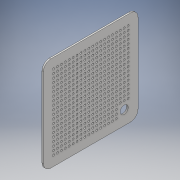
# Autodesk Inventor part: ExtrusionFrontpanel
Saved by Autodesk Inventor 2017 (Build 210142000, 142)
## iProperties
Created: 2019-06-19
Part Number: ExtrusionFrontpanel
Material: Generic
Document SubType Name: Modeling
Designer: DDeGo
Density: 1 g/cm^3
Appearance: Default
Author: DDeGo
Autodesk Inventor part; units mm, degrees
ref_plane "YZ Plane" through (0, 0, 0) normal (1, 0, 0) x (0, 1, 0)
ref_plane "XZ Plane" through (0, 0, 0) normal (0, 1, 0) x (-1, 0, 0)
ref_plane "XY Plane" through (0, 0, 0) normal (0, 0, 1) x (1, 0, 0)
sketch "Sketch1" plane through (0, 0, 0) normal (1, 0, 0) x (0, 1, 0)
  line L0 (0, 15) -> (160, 15)
  line L1 (175, 0) -> (175, -160)
  line L2 (160, -175) -> (0, -175)
  line L3 (-15, -160) -> (-15, 0)
  arc A0 (175, 0) -> (160, 15) centre (160, 0) ccw
  arc A1 (160, -175) -> (175, -160) centre (160, -160) ccw
  arc A2 (-15, -160) -> (0, -175) centre (0, -160) ccw
  arc A3 (0, 15) -> (-15, 0) centre (0, 0) ccw
  point P0 (-15, 15)
  dimension "d0" = 190
  dimension "d1" = 190
  dimension "d4" = 15
  constraints: 8 end point, 8 point on circle, 8 tangent, 4 centre point, 3 equal radius, 2 parallel, 2 point on line, 1 coincident, 1 horizontal, 1 perpendicular
  measures "d0" distance between parallel lines of L2 L0
  measures "d1" distance between parallel lines of L3 L1
  measures "d4" radius of A0
extrude "Extrusion1" add sketch "Sketch1" along normal blind 3
sketch "Sketch2" plane through (3, 0, 0) normal (1, 0, 0) x (0, 0, -1)
  arc A0 (-15, 0) -> (0, -15) centre (0, 0) ccw construction
  arc A1 (0, 175) -> (-15, 160) centre (0, 160) ccw construction
  line L0 (0, 0) -> (0, 160) construction
  line L1 (0, 13) -> (0, 33) construction
  line L2 (4, 13) -> (4, 33)
  line L3 (-4, 33) -> (-4, 13)
  arc A2 (-4, 13) -> (4, 13) centre (0, 13) ccw
  arc A3 (4, 33) -> (-4, 33) centre (0, 33) ccw
  line L4 (0, 51) -> (0, 71) construction
  line L5 (4, 51) -> (4, 71)
  line L6 (-4, 71) -> (-4, 51)
  arc A4 (-4, 51) -> (4, 51) centre (0, 51) ccw
  arc A5 (4, 71) -> (-4, 71) centre (0, 71) ccw
  line L7 (0, 89) -> (0, 109) construction
  line L8 (4, 89) -> (4, 109)
  line L9 (-4, 109) -> (-4, 89)
  arc A6 (-4, 89) -> (4, 89) centre (0, 89) ccw
  arc A7 (4, 109) -> (-4, 109) centre (0, 109) ccw
  line L10 (0, 127) -> (0, 147) construction
  line L11 (4, 127) -> (4, 147)
  line L12 (-4, 147) -> (-4, 127)
  arc A8 (-4, 127) -> (4, 127) centre (0, 127) ccw
  arc A9 (4, 147) -> (-4, 147) centre (0, 147) ccw
  line L13 (0, -15) -> (160, -15) projected
  arc A10 (160, -15) -> (175, 0) centre (160, 0) ccw projected
  line L14 (175, 0) -> (175, 160) projected
  arc A11 (175, 160) -> (160, 175) centre (160, 160) ccw projected
  line L15 (160, 175) -> (0, 175) projected
  arc A12 (0, 175) -> (-15, 160) centre (0, 160) ccw projected
  line L16 (-15, 160) -> (-15, 0) projected
  arc A13 (-15, 0) -> (0, -15) centre (0, 0) ccw projected
  line L17 (0, 0) -> (160, 160) construction
  arc A14 (89, 4) -> (89, -4) centre (89, 0) ccw
  arc A15 (71, -4) -> (71, 4) centre (71, 0) ccw
  line L18 (109, 4) -> (89, 4)
  line L19 (109, 0) -> (89, 0) construction
  line L20 (89, -4) -> (109, -4)
  line L21 (71, 4) -> (51, 4)
  line L22 (71, 0) -> (51, 0) construction
  line L23 (51, -4) -> (71, -4)
  arc A16 (127, 4) -> (127, -4) centre (127, 0) ccw
  arc A17 (33, -4) -> (33, 4) centre (33, 0) ccw
  line L24 (147, 0) -> (127, 0) construction
  line L25 (160, 0) -> (0, 0) construction
  arc A18 (147, -4) -> (147, 4) centre (147, 0) ccw
  line L26 (147, 4) -> (127, 4)
  line L27 (127, -4) -> (147, -4)
  line L28 (33, 4) -> (13, 4)
  line L29 (33, 0) -> (13, 0) construction
  arc A19 (13, 4) -> (13, -4) centre (13, 0) ccw
  arc A20 (109, -4) -> (109, 4) centre (109, 0) ccw
  line L30 (13, -4) -> (33, -4)
  arc A21 (51, 4) -> (51, -4) centre (51, 0) ccw
  arc A22 (156, 89) -> (164, 89) centre (160, 89) ccw
  arc A23 (164, 71) -> (156, 71) centre (160, 71) ccw
  line L31 (156, 109) -> (156, 89)
  line L32 (160, 109) -> (160, 89) construction
  line L33 (164, 89) -> (164, 109)
  line L34 (156, 71) -> (156, 51)
  line L35 (160, 71) -> (160, 51) construction
  line L36 (164, 51) -> (164, 71)
  arc A24 (156, 127) -> (164, 127) centre (160, 127) ccw
  arc A25 (164, 33) -> (156, 33) centre (160, 33) ccw
  line L37 (160, 147) -> (160, 127) construction
  line L38 (160, 160) -> (160, 0) construction
  arc A26 (164, 147) -> (156, 147) centre (160, 147) ccw
  line L39 (156, 147) -> (156, 127)
  line L40 (164, 127) -> (164, 147)
  line L41 (156, 33) -> (156, 13)
  line L42 (160, 33) -> (160, 13) construction
  arc A27 (156, 13) -> (164, 13) centre (160, 13) ccw
  arc A28 (164, 109) -> (156, 109) centre (160, 109) ccw
  line L43 (164, 13) -> (164, 33)
  arc A29 (156, 51) -> (164, 51) centre (160, 51) ccw
  arc A30 (71, 156) -> (71, 164) centre (71, 160) ccw
  arc A31 (89, 164) -> (89, 156) centre (89, 160) ccw
  line L44 (51, 156) -> (71, 156)
  line L45 (51, 160) -> (71, 160) construction
  line L46 (71, 164) -> (51, 164)
  line L47 (89, 156) -> (109, 156)
  line L48 (89, 160) -> (109, 160) construction
  line L49 (109, 164) -> (89, 164)
  arc A32 (33, 156) -> (33, 164) centre (33, 160) ccw
  arc A33 (127, 164) -> (127, 156) centre (127, 160) ccw
  line L50 (13, 160) -> (33, 160) construction
  line L51 (0, 160) -> (160, 160) construction
  arc A34 (13, 164) -> (13, 156) centre (13, 160) ccw
  line L52 (13, 156) -> (33, 156)
  line L53 (33, 164) -> (13, 164)
  line L54 (127, 156) -> (147, 156)
  line L55 (127, 160) -> (147, 160) construction
  arc A35 (147, 156) -> (147, 164) centre (147, 160) ccw
  arc A36 (51, 164) -> (51, 156) centre (51, 160) ccw
  line L56 (147, 164) -> (127, 164)
  arc A37 (109, 156) -> (109, 164) centre (109, 160) ccw
  point P0 (0, 23)
  point P1 (0, 61)
  point P2 (0, 99)
  point P3 (0, 137)
  point P4 (80, 80)
  point P5 (99, 0)
  point P6 (61, 0)
  point P7 (137, 0)
  point P8 (23, 0)
  point P9 (160, 99)
  point P10 (160, 61)
  point P11 (160, 137)
  point P12 (160, 23)
  point P13 (61, 160)
  point P14 (99, 160)
  point P15 (23, 160)
  point P16 (137, 160)
  dimension "d7" = 13
  dimension "d8" = 4
  dimension "d9" = 20
  dimension "d12" = 38
  dimension "d20" = 360
  dimension "d24" = 13
  constraints: 138 end point, 64 point on circle, 32 centre point, 8 point on line, 4 tangent, 2 midpoint, 2 vertical, 1 parallel, 253 other
  measures "d7" distance of point (0, 0) L1.start
  measures "d8" radius of A2
  measures "d9" distance of L1.end L1.start
  measures "d12" distance of L2.start L5.start
  measures "d24" distance of point (0, 160) L10.end
extrude "perimeterslots" [suppressed]
sketch "Sketch3" plane through (3, 0, 0) normal (1, 0, 0) x (0, 0, -1)
  circle A0 centre (155, 5) radius 2
  line L0 (175, 0) -> (175, 160) projected
  line L1 (0, -15) -> (160, -15) projected
  circle A1 centre (155, 12.8947) radius 2
  circle A2 centre (155, 20.7895) radius 2
  circle A3 centre (155, 28.6842) radius 2
  circle A4 centre (155, 36.5789) radius 2
  circle A5 centre (155, 44.4737) radius 2
  circle A6 centre (155, 52.3684) radius 2
  circle A7 centre (155, 60.2632) radius 2
  circle A8 centre (155, 68.1579) radius 2
  circle A9 centre (155, 76.0526) radius 2
  circle A10 centre (155, 83.9474) radius 2
  circle A11 centre (155, 91.8421) radius 2
  circle A12 centre (155, 99.7368) radius 2
  circle A13 centre (155, 107.6316) radius 2
  circle A14 centre (155, 115.5263) radius 2
  circle A15 centre (155, 123.4211) radius 2
  circle A16 centre (155, 131.3158) radius 2
  circle A17 centre (155, 139.2105) radius 2
  circle A18 centre (155, 147.1053) radius 2
  circle A19 centre (155, 155) radius 2
  circle A20 centre (147.1053, 5) radius 2
  circle A21 centre (147.1053, 12.8947) radius 2
  circle A22 centre (147.1053, 20.7895) radius 2
  circle A23 centre (147.1053, 28.6842) radius 2
  circle A24 centre (147.1053, 36.5789) radius 2
  circle A25 centre (147.1053, 44.4737) radius 2
  circle A26 centre (147.1053, 52.3684) radius 2
  circle A27 centre (147.1053, 60.2632) radius 2
  circle A28 centre (147.1053, 68.1579) radius 2
  circle A29 centre (147.1053, 76.0526) radius 2
  circle A30 centre (147.1053, 83.9474) radius 2
  circle A31 centre (147.1053, 91.8421) radius 2
  circle A32 centre (147.1053, 99.7368) radius 2
  circle A33 centre (147.1053, 107.6316) radius 2
  circle A34 centre (147.1053, 115.5263) radius 2
  circle A35 centre (147.1053, 123.4211) radius 2
  circle A36 centre (147.1053, 131.3158) radius 2
  circle A37 centre (147.1053, 139.2105) radius 2
  circle A38 centre (147.1053, 147.1053) radius 2
  circle A39 centre (147.1053, 155) radius 2
  circle A40 centre (139.2105, 5) radius 2
  circle A41 centre (139.2105, 12.8947) radius 2
  circle A42 centre (139.2105, 20.7895) radius 2
  circle A43 centre (139.2105, 28.6842) radius 2
  circle A44 centre (139.2105, 36.5789) radius 2
  circle A45 centre (139.2105, 44.4737) radius 2
  circle A46 centre (139.2105, 52.3684) radius 2
  circle A47 centre (139.2105, 60.2632) radius 2
  circle A48 centre (139.2105, 68.1579) radius 2
  circle A49 centre (139.2105, 76.0526) radius 2
  circle A50 centre (139.2105, 83.9474) radius 2
  circle A51 centre (139.2105, 91.8421) radius 2
  circle A52 centre (139.2105, 99.7368) radius 2
  circle A53 centre (139.2105, 107.6316) radius 2
  circle A54 centre (139.2105, 115.5263) radius 2
  circle A55 centre (139.2105, 123.4211) radius 2
  circle A56 centre (139.2105, 131.3158) radius 2
  circle A57 centre (139.2105, 139.2105) radius 2
  circle A58 centre (139.2105, 147.1053) radius 2
  circle A59 centre (139.2105, 155) radius 2
  circle A60 centre (131.3158, 5) radius 2
  circle A61 centre (131.3158, 12.8947) radius 2
  circle A62 centre (131.3158, 20.7895) radius 2
  circle A63 centre (131.3158, 28.6842) radius 2
  circle A64 centre (131.3158, 36.5789) radius 2
  circle A65 centre (131.3158, 44.4737) radius 2
  circle A66 centre (131.3158, 52.3684) radius 2
  circle A67 centre (131.3158, 60.2632) radius 2
  circle A68 centre (131.3158, 68.1579) radius 2
  circle A69 centre (131.3158, 76.0526) radius 2
  circle A70 centre (131.3158, 83.9474) radius 2
  circle A71 centre (131.3158, 91.8421) radius 2
  circle A72 centre (131.3158, 99.7368) radius 2
  circle A73 centre (131.3158, 107.6316) radius 2
  circle A74 centre (131.3158, 115.5263) radius 2
  circle A75 centre (131.3158, 123.4211) radius 2
  circle A76 centre (131.3158, 131.3158) radius 2
  circle A77 centre (131.3158, 139.2105) radius 2
  circle A78 centre (131.3158, 147.1053) radius 2
  circle A79 centre (131.3158, 155) radius 2
  circle A80 centre (123.4211, 5) radius 2
  circle A81 centre (123.4211, 12.8947) radius 2
  circle A82 centre (123.4211, 20.7895) radius 2
  circle A83 centre (123.4211, 28.6842) radius 2
  circle A84 centre (123.4211, 36.5789) radius 2
  circle A85 centre (123.4211, 44.4737) radius 2
  circle A86 centre (123.4211, 52.3684) radius 2
  circle A87 centre (123.4211, 60.2632) radius 2
  circle A88 centre (123.4211, 68.1579) radius 2
  circle A89 centre (123.4211, 76.0526) radius 2
  circle A90 centre (123.4211, 83.9474) radius 2
  circle A91 centre (123.4211, 91.8421) radius 2
  circle A92 centre (123.4211, 99.7368) radius 2
  circle A93 centre (123.4211, 107.6316) radius 2
  circle A94 centre (123.4211, 115.5263) radius 2
  circle A95 centre (123.4211, 123.4211) radius 2
  circle A96 centre (123.4211, 131.3158) radius 2
  circle A97 centre (123.4211, 139.2105) radius 2
  circle A98 centre (123.4211, 147.1053) radius 2
  circle A99 centre (123.4211, 155) radius 2
  circle A100 centre (115.5263, 5) radius 2
  circle A101 centre (115.5263, 12.8947) radius 2
  circle A102 centre (115.5263, 20.7895) radius 2
  circle A103 centre (115.5263, 28.6842) radius 2
  circle A104 centre (115.5263, 36.5789) radius 2
  circle A105 centre (115.5263, 44.4737) radius 2
  circle A106 centre (115.5263, 52.3684) radius 2
  circle A107 centre (115.5263, 60.2632) radius 2
  circle A108 centre (115.5263, 68.1579) radius 2
  circle A109 centre (115.5263, 76.0526) radius 2
  circle A110 centre (115.5263, 83.9474) radius 2
  circle A111 centre (115.5263, 91.8421) radius 2
  circle A112 centre (115.5263, 99.7368) radius 2
  circle A113 centre (115.5263, 107.6316) radius 2
  circle A114 centre (115.5263, 115.5263) radius 2
  circle A115 centre (115.5263, 123.4211) radius 2
  circle A116 centre (115.5263, 131.3158) radius 2
  circle A117 centre (115.5263, 139.2105) radius 2
  circle A118 centre (115.5263, 147.1053) radius 2
  circle A119 centre (115.5263, 155) radius 2
  circle A120 centre (107.6316, 5) radius 2
  circle A121 centre (107.6316, 12.8947) radius 2
  circle A122 centre (107.6316, 20.7895) radius 2
  circle A123 centre (107.6316, 28.6842) radius 2
  circle A124 centre (107.6316, 36.5789) radius 2
  circle A125 centre (107.6316, 44.4737) radius 2
  circle A126 centre (107.6316, 52.3684) radius 2
  circle A127 centre (107.6316, 60.2632) radius 2
  circle A128 centre (107.6316, 68.1579) radius 2
  circle A129 centre (107.6316, 76.0526) radius 2
  circle A130 centre (107.6316, 83.9474) radius 2
  circle A131 centre (107.6316, 91.8421) radius 2
  circle A132 centre (107.6316, 99.7368) radius 2
  circle A133 centre (107.6316, 107.6316) radius 2
  circle A134 centre (107.6316, 115.5263) radius 2
  circle A135 centre (107.6316, 123.4211) radius 2
  circle A136 centre (107.6316, 131.3158) radius 2
  circle A137 centre (107.6316, 139.2105) radius 2
  circle A138 centre (107.6316, 147.1053) radius 2
  circle A139 centre (107.6316, 155) radius 2
  circle A140 centre (99.7368, 5) radius 2
  circle A141 centre (99.7368, 12.8947) radius 2
  circle A142 centre (99.7368, 20.7895) radius 2
  circle A143 centre (99.7368, 28.6842) radius 2
  circle A144 centre (99.7368, 36.5789) radius 2
  circle A145 centre (99.7368, 44.4737) radius 2
  circle A146 centre (99.7368, 52.3684) radius 2
  circle A147 centre (99.7368, 60.2632) radius 2
  circle A148 centre (99.7368, 68.1579) radius 2
  circle A149 centre (99.7368, 76.0526) radius 2
  circle A150 centre (99.7368, 83.9474) radius 2
  circle A151 centre (99.7368, 91.8421) radius 2
  circle A152 centre (99.7368, 99.7368) radius 2
  circle A153 centre (99.7368, 107.6316) radius 2
  circle A154 centre (99.7368, 115.5263) radius 2
  circle A155 centre (99.7368, 123.4211) radius 2
  circle A156 centre (99.7368, 131.3158) radius 2
  circle A157 centre (99.7368, 139.2105) radius 2
  circle A158 centre (99.7368, 147.1053) radius 2
  circle A159 centre (99.7368, 155) radius 2
  circle A160 centre (91.8421, 5) radius 2
  circle A161 centre (91.8421, 12.8947) radius 2
  circle A162 centre (91.8421, 20.7895) radius 2
  circle A163 centre (91.8421, 28.6842) radius 2
  circle A164 centre (91.8421, 36.5789) radius 2
  circle A165 centre (91.8421, 44.4737) radius 2
  circle A166 centre (91.8421, 52.3684) radius 2
  circle A167 centre (91.8421, 60.2632) radius 2
  circle A168 centre (91.8421, 68.1579) radius 2
  circle A169 centre (91.8421, 76.0526) radius 2
  circle A170 centre (91.8421, 83.9474) radius 2
  circle A171 centre (91.8421, 91.8421) radius 2
  circle A172 centre (91.8421, 99.7368) radius 2
  circle A173 centre (91.8421, 107.6316) radius 2
  circle A174 centre (91.8421, 115.5263) radius 2
  circle A175 centre (91.8421, 123.4211) radius 2
  circle A176 centre (91.8421, 131.3158) radius 2
  circle A177 centre (91.8421, 139.2105) radius 2
  circle A178 centre (91.8421, 147.1053) radius 2
  circle A179 centre (91.8421, 155) radius 2
  circle A180 centre (83.9474, 5) radius 2
  circle A181 centre (83.9474, 12.8947) radius 2
  circle A182 centre (83.9474, 20.7895) radius 2
  circle A183 centre (83.9474, 28.6842) radius 2
  circle A184 centre (83.9474, 36.5789) radius 2
  circle A185 centre (83.9474, 44.4737) radius 2
  circle A186 centre (83.9474, 52.3684) radius 2
  circle A187 centre (83.9474, 60.2632) radius 2
  circle A188 centre (83.9474, 68.1579) radius 2
  circle A189 centre (83.9474, 76.0526) radius 2
  circle A190 centre (83.9474, 83.9474) radius 2
  circle A191 centre (83.9474, 91.8421) radius 2
  circle A192 centre (83.9474, 99.7368) radius 2
  circle A193 centre (83.9474, 107.6316) radius 2
  circle A194 centre (83.9474, 115.5263) radius 2
  circle A195 centre (83.9474, 123.4211) radius 2
  circle A196 centre (83.9474, 131.3158) radius 2
  circle A197 centre (83.9474, 139.2105) radius 2
  circle A198 centre (83.9474, 147.1053) radius 2
  circle A199 centre (83.9474, 155) radius 2
  circle A200 centre (76.0526, 5) radius 2
  circle A201 centre (76.0526, 12.8947) radius 2
  circle A202 centre (76.0526, 20.7895) radius 2
  circle A203 centre (76.0526, 28.6842) radius 2
  circle A204 centre (76.0526, 36.5789) radius 2
  circle A205 centre (76.0526, 44.4737) radius 2
  circle A206 centre (76.0526, 52.3684) radius 2
  circle A207 centre (76.0526, 60.2632) radius 2
  circle A208 centre (76.0526, 68.1579) radius 2
  circle A209 centre (76.0526, 76.0526) radius 2
  circle A210 centre (76.0526, 83.9474) radius 2
  circle A211 centre (76.0526, 91.8421) radius 2
  circle A212 centre (76.0526, 99.7368) radius 2
  circle A213 centre (76.0526, 107.6316) radius 2
  circle A214 centre (76.0526, 115.5263) radius 2
  circle A215 centre (76.0526, 123.4211) radius 2
  circle A216 centre (76.0526, 131.3158) radius 2
  circle A217 centre (76.0526, 139.2105) radius 2
  circle A218 centre (76.0526, 147.1053) radius 2
  circle A219 centre (76.0526, 155) radius 2
  circle A220 centre (68.1579, 5) radius 2
  circle A221 centre (68.1579, 12.8947) radius 2
  circle A222 centre (68.1579, 20.7895) radius 2
  circle A223 centre (68.1579, 28.6842) radius 2
  circle A224 centre (68.1579, 36.5789) radius 2
  circle A225 centre (68.1579, 44.4737) radius 2
  circle A226 centre (68.1579, 52.3684) radius 2
  circle A227 centre (68.1579, 60.2632) radius 2
  circle A228 centre (68.1579, 68.1579) radius 2
  circle A229 centre (68.1579, 76.0526) radius 2
  circle A230 centre (68.1579, 83.9474) radius 2
  circle A231 centre (68.1579, 91.8421) radius 2
  circle A232 centre (68.1579, 99.7368) radius 2
  circle A233 centre (68.1579, 107.6316) radius 2
  circle A234 centre (68.1579, 115.5263) radius 2
  circle A235 centre (68.1579, 123.4211) radius 2
  circle A236 centre (68.1579, 131.3158) radius 2
  circle A237 centre (68.1579, 139.2105) radius 2
  circle A238 centre (68.1579, 147.1053) radius 2
  circle A239 centre (68.1579, 155) radius 2
  circle A240 centre (60.2632, 5) radius 2
  circle A241 centre (60.2632, 12.8947) radius 2
  circle A242 centre (60.2632, 20.7895) radius 2
  circle A243 centre (60.2632, 28.6842) radius 2
  circle A244 centre (60.2632, 36.5789) radius 2
  circle A245 centre (60.2632, 44.4737) radius 2
  circle A246 centre (60.2632, 52.3684) radius 2
  circle A247 centre (60.2632, 60.2632) radius 2
  circle A248 centre (60.2632, 68.1579) radius 2
  circle A249 centre (60.2632, 76.0526) radius 2
  circle A250 centre (60.2632, 83.9474) radius 2
  circle A251 centre (60.2632, 91.8421) radius 2
  circle A252 centre (60.2632, 99.7368) radius 2
  circle A253 centre (60.2632, 107.6316) radius 2
  circle A254 centre (60.2632, 115.5263) radius 2
  circle A255 centre (60.2632, 123.4211) radius 2
  circle A256 centre (60.2632, 131.3158) radius 2
  circle A257 centre (60.2632, 139.2105) radius 2
  circle A258 centre (60.2632, 147.1053) radius 2
  circle A259 centre (60.2632, 155) radius 2
  circle A260 centre (52.3684, 5) radius 2
  circle A261 centre (52.3684, 12.8947) radius 2
  circle A262 centre (52.3684, 20.7895) radius 2
  circle A263 centre (52.3684, 28.6842) radius 2
  circle A264 centre (52.3684, 36.5789) radius 2
  circle A265 centre (52.3684, 44.4737) radius 2
  circle A266 centre (52.3684, 52.3684) radius 2
  circle A267 centre (52.3684, 60.2632) radius 2
  circle A268 centre (52.3684, 68.1579) radius 2
  circle A269 centre (52.3684, 76.0526) radius 2
  circle A270 centre (52.3684, 83.9474) radius 2
  circle A271 centre (52.3684, 91.8421) radius 2
  circle A272 centre (52.3684, 99.7368) radius 2
  circle A273 centre (52.3684, 107.6316) radius 2
  circle A274 centre (52.3684, 115.5263) radius 2
  circle A275 centre (52.3684, 123.4211) radius 2
  circle A276 centre (52.3684, 131.3158) radius 2
  circle A277 centre (52.3684, 139.2105) radius 2
  circle A278 centre (52.3684, 147.1053) radius 2
  circle A279 centre (52.3684, 155) radius 2
  circle A280 centre (44.4737, 5) radius 2
  circle A281 centre (44.4737, 12.8947) radius 2
  circle A282 centre (44.4737, 20.7895) radius 2
  circle A283 centre (44.4737, 28.6842) radius 2
  circle A284 centre (44.4737, 36.5789) radius 2
  circle A285 centre (44.4737, 44.4737) radius 2
  circle A286 centre (44.4737, 52.3684) radius 2
  circle A287 centre (44.4737, 60.2632) radius 2
  circle A288 centre (44.4737, 68.1579) radius 2
  circle A289 centre (44.4737, 76.0526) radius 2
  circle A290 centre (44.4737, 83.9474) radius 2
  circle A291 centre (44.4737, 91.8421) radius 2
  circle A292 centre (44.4737, 99.7368) radius 2
  circle A293 centre (44.4737, 107.6316) radius 2
  circle A294 centre (44.4737, 115.5263) radius 2
  circle A295 centre (44.4737, 123.4211) radius 2
  circle A296 centre (44.4737, 131.3158) radius 2
  circle A297 centre (44.4737, 139.2105) radius 2
  circle A298 centre (44.4737, 147.1053) radius 2
  circle A299 centre (44.4737, 155) radius 2
  circle A300 centre (36.5789, 5) radius 2
  circle A301 centre (36.5789, 12.8947) radius 2
  circle A302 centre (36.5789, 20.7895) radius 2
  circle A303 centre (36.5789, 28.6842) radius 2
  circle A304 centre (36.5789, 36.5789) radius 2
  circle A305 centre (36.5789, 44.4737) radius 2
  circle A306 centre (36.5789, 52.3684) radius 2
  circle A307 centre (36.5789, 60.2632) radius 2
  circle A308 centre (36.5789, 68.1579) radius 2
  circle A309 centre (36.5789, 76.0526) radius 2
  circle A310 centre (36.5789, 83.9474) radius 2
  circle A311 centre (36.5789, 91.8421) radius 2
  circle A312 centre (36.5789, 99.7368) radius 2
  circle A313 centre (36.5789, 107.6316) radius 2
  circle A314 centre (36.5789, 115.5263) radius 2
  circle A315 centre (36.5789, 123.4211) radius 2
  circle A316 centre (36.5789, 131.3158) radius 2
  circle A317 centre (36.5789, 139.2105) radius 2
  circle A318 centre (36.5789, 147.1053) radius 2
  circle A319 centre (36.5789, 155) radius 2
  circle A320 centre (28.6842, 5) radius 2
  circle A321 centre (28.6842, 12.8947) radius 2
  circle A322 centre (28.6842, 20.7895) radius 2
  circle A323 centre (28.6842, 28.6842) radius 2
  circle A324 centre (28.6842, 36.5789) radius 2
  circle A325 centre (28.6842, 44.4737) radius 2
  circle A326 centre (28.6842, 52.3684) radius 2
  circle A327 centre (28.6842, 60.2632) radius 2
  circle A328 centre (28.6842, 68.1579) radius 2
  circle A329 centre (28.6842, 76.0526) radius 2
  circle A330 centre (28.6842, 83.9474) radius 2
  circle A331 centre (28.6842, 91.8421) radius 2
  circle A332 centre (28.6842, 99.7368) radius 2
  circle A333 centre (28.6842, 107.6316) radius 2
  circle A334 centre (28.6842, 115.5263) radius 2
  circle A335 centre (28.6842, 123.4211) radius 2
  circle A336 centre (28.6842, 131.3158) radius 2
  circle A337 centre (28.6842, 139.2105) radius 2
  circle A338 centre (28.6842, 147.1053) radius 2
  circle A339 centre (28.6842, 155) radius 2
  circle A340 centre (20.7895, 5) radius 2
  circle A341 centre (20.7895, 12.8947) radius 2
  circle A342 centre (20.7895, 20.7895) radius 2
  circle A343 centre (20.7895, 28.6842) radius 2
  circle A344 centre (20.7895, 36.5789) radius 2
  circle A345 centre (20.7895, 44.4737) radius 2
  circle A346 centre (20.7895, 52.3684) radius 2
  circle A347 centre (20.7895, 60.2632) radius 2
  circle A348 centre (20.7895, 68.1579) radius 2
  circle A349 centre (20.7895, 76.0526) radius 2
  circle A350 centre (20.7895, 83.9474) radius 2
  circle A351 centre (20.7895, 91.8421) radius 2
  circle A352 centre (20.7895, 99.7368) radius 2
  circle A353 centre (20.7895, 107.6316) radius 2
  circle A354 centre (20.7895, 115.5263) radius 2
  circle A355 centre (20.7895, 123.4211) radius 2
  circle A356 centre (20.7895, 131.3158) radius 2
  circle A357 centre (20.7895, 139.2105) radius 2
  circle A358 centre (20.7895, 147.1053) radius 2
  circle A359 centre (20.7895, 155) radius 2
  circle A360 centre (12.8947, 5) radius 2
  circle A361 centre (12.8947, 12.8947) radius 2
  circle A362 centre (12.8947, 20.7895) radius 2
  circle A363 centre (12.8947, 28.6842) radius 2
  circle A364 centre (12.8947, 36.5789) radius 2
  circle A365 centre (12.8947, 44.4737) radius 2
  circle A366 centre (12.8947, 52.3684) radius 2
  circle A367 centre (12.8947, 60.2632) radius 2
  circle A368 centre (12.8947, 68.1579) radius 2
  circle A369 centre (12.8947, 76.0526) radius 2
  circle A370 centre (12.8947, 83.9474) radius 2
  circle A371 centre (12.8947, 91.8421) radius 2
  circle A372 centre (12.8947, 99.7368) radius 2
  circle A373 centre (12.8947, 107.6316) radius 2
  circle A374 centre (12.8947, 115.5263) radius 2
  circle A375 centre (12.8947, 123.4211) radius 2
  circle A376 centre (12.8947, 131.3158) radius 2
  circle A377 centre (12.8947, 139.2105) radius 2
  circle A378 centre (12.8947, 147.1053) radius 2
  circle A379 centre (12.8947, 155) radius 2
  circle A380 centre (5, 5) radius 2
  circle A381 centre (5, 12.8947) radius 2
  circle A382 centre (5, 20.7895) radius 2
  circle A383 centre (5, 28.6842) radius 2
  circle A384 centre (5, 36.5789) radius 2
  circle A385 centre (5, 44.4737) radius 2
  circle A386 centre (5, 52.3684) radius 2
  circle A387 centre (5, 60.2632) radius 2
  circle A388 centre (5, 68.1579) radius 2
  circle A389 centre (5, 76.0526) radius 2
  circle A390 centre (5, 83.9474) radius 2
  circle A391 centre (5, 91.8421) radius 2
  circle A392 centre (5, 99.7368) radius 2
  circle A393 centre (5, 107.6316) radius 2
  circle A394 centre (5, 115.5263) radius 2
  circle A395 centre (5, 123.4211) radius 2
  circle A396 centre (5, 131.3158) radius 2
  circle A397 centre (5, 139.2105) radius 2
  circle A398 centre (5, 147.1053) radius 2
  circle A399 centre (5, 155) radius 2
  line L2 (160, 175) -> (0, 175) projected
  line L3 (-15, 160) -> (-15, 0) projected
  point P0 (0, 0)
  dimension "d25" = 20
  dimension "d26" = 20
  dimension "d27" = 4
  dimension "d30" = 7.8947
  dimension "d33" = 7.8947
  dimension "d36" = 20
  dimension "d37" = 20
  constraints: 400 centre point, 1 horizontal, 1 vertical, 798 other
  measures "d25" distance from line of A0.centre L0
  measures "d26" distance from line of L1 A0.centre
  measures "d27" diameter of A0
  measures "d30" distance of A0.centre A1.centre
  measures "d33" distance of A0.centre A20.centre
  measures "d36" distance from line of L2 A19.centre
  measures "d37" distance from line of L3 A380.centre
extrude "dotarray" cut sketch "Sketch3" against normal blind 10 contours A0 | A1 | A2 | A3 | A4 | A5 | A6 | A7 | A8 | A9 | A10 | A11 | A12 | A13 | A14 | A15 | A16 | A20 | A21 | A22 | A23 | A24 | A25 | A26 | A27 | A28 | A29 | A30 | A31 | A32 | A33 | A34 | A35 | A36 | A40 | A41 | A42 | A43 | A44 | A45 | A46 | A47 | A48 | A49 | A50 | A51 | A52 | A53 | A54 | A55 | A56 | A60 | A61 | A62 | A63 | A64 | A65 | A66 | A67 | A68 | A69 | A70 | A71 | A72 | A73 | A74 | A75 | A76 | A77 | A78 | A79 | A80 | A81 | A82 | A83 | A84 | A85 | A86 | A87 | A88 | A89 | A90 | A91 | A92 | A93 | A94 | A95 | A96 | A97 | A98 | A99 | A100 | A101 | A102 | A103 | A104 | A105 | A106 | A107 | A108 | A109 | A110 | A111 | A112 | A113 | A114 | A115 | A116 | A117 | A118 | A119 | A120 | A121 | A122 | A123 | A124 | A125 | A126 | A127 | A128 | A129 | A130 | A131 | A132 | A133 | A134 | A135 | A136 | A137 | A138 | A139 | A140 | A141 | A142 | A143 | A144 | A145 | A146 | A147 | A148 | A149 | A150 | A151 | A152 | A153 | A154 | A155 | A156 | A157 | A158 | A159 | A160 | A161 | A162 | A163 | A164 | A165 | A166 | A167 | A168 | A169 | A170 | A171 | A172 | A173 | A174 | A175 | A176 | A177 | A178 | A179 | A180 | A181 | A182 | A183 | A184 | A185 | A186 | A187 | A188 | A189 | A190 | A191 | A192 | A193 | A194 | A195 | A196 | A197 | A198 | A199 | A200 | A201 | A202 | A203 | A204 | A205 | A206 | A207 | A208 | A209 | A210 | A211 | A212 | A213 | A214 | A215 | A216 | A217 | A218 | A219 | A220 | A221 | A222 | A223 | A224 | A225 | A226 | A227 | A228 | A229 | A230 | A231 | A232 | A233 | A234 | A235 | A236 | A237 | A238 | A239 | A240 | A241 | A242 | A243 | A244 | A245 | A246 | A247 | A248 | A249 | A250 | A251 | A252 | A253 | A254 | A255 | A256 | A257 | A258 | A259 | A260 | A261 | A262 | A263 | A264 | A265 | A266 | A267 | A268 | A269 | A270 | A271 | A272 | A273 | A274 | A275 | A276 | A277 | A278 | A279 | A280 | A281 | A282 | A283 | A284 | A285 | A286 | A287 | A288 | A289 | A290 | A291 | A292 | A293 | A294 | A295 | A296 | A297 | A298 | A299 | A300 | A301 | A302 | A303 | A304 | A305 | A306 | A307 | A308 | A309 | A310 | A311 | A312 | A313 | A314 | A315 | A316 | A317 | A318 | A319 | A320 | A321 | A322 | A323 | A324 | A325 | A326 | A327 | A328 | A329 | A330 | A331 | A332 | A333 | A334 | A335 | A336 | A337 | A338 | A339 | A340 | A341 | A342 | A343 | A344 | A345 | A346 | A347 | A348 | A349 | A350 | A351 | A352 | A353 | A354 | A355 | A356 | A357 | A358 | A359 | A360 | A361 | A362 | A363 | A364 | A365 | A366 | A367 | A368 | A369 | A370 | A371 | A372 | A373 | A374 | A375 | A376 | A377 | A378 | A379 | A380 | A381 | A382 | A383 | A384 | A385 | A386 | A387 | A388 | A389 | A390 | A391 | A392 | A393 | A394 | A395 | A396 | A397 | A398 | A399
sketch "Sketch4" plane through (3, 0, 0) normal (1, 0, 0) x (0, 0, -1)
  circle A0 centre (147.1053, 147.1053) radius 8.1
  circle A1 centre (147.1053, 131.3158) radius 2 projected
  line L0 (147.1053, 131.3158) -> (147.1053, 147.1053) construction
  circle A2 centre (131.3158, 147.1053) radius 2 projected
  line L1 (147.1053, 147.1053) -> (131.3158, 147.1053) construction
  point P0 (0, 0)
  dimension "d40" = 16.2
  constraints: 4 end point, 1 centre point, 1 coincident, 1 horizontal, 1 vertical
  measures "d40" diameter of A0
extrude "Extrusion4" cut sketch "Sketch4" against normal blind 10 contours A0
equation "\"d24\" = d7"
body "Solid1"
